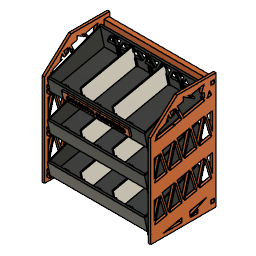
binstack-print-assembly (Autodesk Fusion 360 design; units mm, degrees)
part number: 2026-08-18-20-49-02-766
part number: 2026-08-18-20-49-04-076
part number: 2026-08-18-20-49-04-669
part number: 2026-08-18-20-49-05-390
part number: 2026-08-18-20-49-06-631
part number: 2026-08-18-20-49-07-047
part number: 2026-08-18-20-49-07-130
Autodesk Fusion 360 part; units mm, degrees
sketch "Sketch1" plane through (0, 0, 0) normal (1, 0, 0) x (0, 0, -1) in component "Боковина левая"
  line L0 (0, 15) -> (0, 150)
  line L1 (0, 150) -> (-240, 150)
  line L2 (-240, 150) -> (-240, 70)
  line L3 (-240, 70) -> (-190, 15)
  line L4 (-190, 15) -> (0, 15)
extrude "Extrude1" add sketch "Sketch1" along normal blind 5 from surface at 3 makes body 1 in component "Боковина левая"
sketch "Sketch2" plane through (0, 0, 0) normal (1, 0, 0) x (0, 0, -1) in component "Боковина левая"
  line L0 (-9, 20) -> (-35.5696, 145)
  line L1 (-35.5696, 145) -> (-41.5696, 145)
  line L2 (-41.5696, 145) -> (-15, 20)
  line L3 (-15, 20) -> (-9, 20)
extrude "Extrude2" add sketch "Sketch2" along normal blind 6 from surface at 8 separate body makes body 2 in component "Боковина левая"
sketch "Sketch3" plane through (0, 0, 0) normal (1, 0, 0) x (0, 0, -1) in component "Боковина левая"
  line L0 (-18.2, 20) -> (-44.7696, 145)
  line L1 (-44.7696, 145) -> (-49.7696, 145)
  line L2 (-49.7696, 145) -> (-23.2, 20)
  line L3 (-23.2, 20) -> (-18.2, 20)
extrude "Extrude3" add sketch "Sketch3" along normal blind 6 from surface at 8 separate body makes body 3 in component "Боковина левая"
sketch "Sketch4" plane through (0, 0, 0) normal (1, 0, 0) x (0, 0, -1) in component "Боковина левая"
  line L0 (-16.2753, 26) -> (-17.2753, 28)
  line L1 (-17.2753, 28) -> (-18.3381, 31)
  line L2 (-18.3381, 31) -> (-17.7632, 33)
  line L3 (-17.7632, 33) -> (-16.2753, 26)
extrude "Extrude4" add sketch "Sketch4" along normal blind 6 from surface at 8 separate body makes body 4 in component "Боковина левая"
sketch "Sketch5" plane through (0, 0, 0) normal (1, 0, 0) x (0, 0, -1) in component "Боковина левая"
  line L0 (-84, 20) -> (-110.5696, 145)
  line L1 (-110.5696, 145) -> (-116.5696, 145)
  line L2 (-116.5696, 145) -> (-90, 20)
  line L3 (-90, 20) -> (-84, 20)
extrude "Extrude5" add sketch "Sketch5" along normal blind 6 from surface at 8 separate body makes body 5 in component "Боковина левая"
sketch "Sketch6" plane through (0, 0, 0) normal (1, 0, 0) x (0, 0, -1) in component "Боковина левая"
  line L0 (-93.2, 20) -> (-119.7696, 145)
  line L1 (-119.7696, 145) -> (-124.7696, 145)
  line L2 (-124.7696, 145) -> (-98.2, 20)
  line L3 (-98.2, 20) -> (-93.2, 20)
extrude "Extrude6" add sketch "Sketch6" along normal blind 6 from surface at 8 separate body makes body 6 in component "Боковина левая"
sketch "Sketch7" plane through (0, 0, 0) normal (1, 0, 0) x (0, 0, -1) in component "Боковина левая"
  line L0 (-91.2753, 26) -> (-92.2753, 28)
  line L1 (-92.2753, 28) -> (-93.3381, 31)
  line L2 (-93.3381, 31) -> (-92.7632, 33)
  line L3 (-92.7632, 33) -> (-91.2753, 26)
extrude "Extrude7" add sketch "Sketch7" along normal blind 6 from surface at 8 separate body makes body 7 in component "Боковина левая"
sketch "Sketch8" plane through (0, 0, 0) normal (1, 0, 0) x (0, 0, -1) in component "Боковина левая"
  line L0 (-159, 20) -> (-185.5696, 145)
  line L1 (-185.5696, 145) -> (-191.5696, 145)
  line L2 (-191.5696, 145) -> (-165, 20)
  line L3 (-165, 20) -> (-159, 20)
extrude "Extrude8" add sketch "Sketch8" along normal blind 6 from surface at 8 separate body makes body 8 in component "Боковина левая"
sketch "Sketch9" plane through (0, 0, 0) normal (1, 0, 0) x (0, 0, -1) in component "Боковина левая"
  line L0 (-168.2, 20) -> (-194.7696, 145)
  line L1 (-194.7696, 145) -> (-199.7696, 145)
  line L2 (-199.7696, 145) -> (-173.2, 20)
  line L3 (-173.2, 20) -> (-168.2, 20)
extrude "Extrude9" add sketch "Sketch9" along normal blind 6 from surface at 8 separate body makes body 9 in component "Боковина левая"
sketch "Sketch10" plane through (0, 0, 0) normal (1, 0, 0) x (0, 0, -1) in component "Боковина левая"
  line L0 (-166.2753, 26) -> (-167.2753, 28)
  line L1 (-167.2753, 28) -> (-168.3381, 31)
  line L2 (-168.3381, 31) -> (-167.7632, 33)
  line L3 (-167.7632, 33) -> (-166.2753, 26)
extrude "Extrude10" add sketch "Sketch10" along normal blind 6 from surface at 8 separate body makes body 10 in component "Боковина левая"
combine "Combine1" operation add target body 1 tool bodies 2 3 4 5 6 7 8 9 10 in component "Боковина левая"
sketch "Sketch11" plane through (0, 0, 0) normal (1, 0, 0) x (0, 0, -1) in component "Боковина левая"
  line L0 (-10.5, 139.5) -> (-10.5, 146.5)
  line L1 (-10.5, 146.5) -> (-17.5, 146.5)
  line L2 (-17.5, 146.5) -> (-17.5, 139.5)
  line L3 (-17.5, 139.5) -> (-10.5, 139.5)
extrude "Extrude11" cut sketch "Sketch11" along normal blind 30 from surface at -2 bodies 1 in component "Боковина левая"
sketch "Sketch12" plane through (0, 0, 0) normal (1, 0, 0) x (0, 0, -1) in component "Боковина левая"
  line L0 (-222.5, 139.5) -> (-222.5, 146.5)
  line L1 (-222.5, 146.5) -> (-229.5, 146.5)
  line L2 (-229.5, 146.5) -> (-229.5, 139.5)
  line L3 (-229.5, 139.5) -> (-222.5, 139.5)
extrude "Extrude12" cut sketch "Sketch12" along normal blind 30 from surface at -2 bodies 1 in component "Боковина левая"
sketch "Sketch13" plane through (0, 0, 0) normal (1, 0, 0) x (0, 0, -1) in component "Боковина левая"
  line L0 (-31.0484, 23.6788) -> (-36.4457, 49.0712)
  line L1 (-36.4457, 49.0712) -> (-77.3478, 36.375)
  line L2 (-77.3478, 36.375) -> (-31.0484, 23.6788)
  line L3 (-37.5845, 54.4288) -> (-42.9818, 79.8212)
  line L4 (-42.9818, 79.8212) -> (-83.8839, 67.125)
  line L5 (-83.8839, 67.125) -> (-37.5845, 54.4288)
  line L6 (-44.1206, 85.1788) -> (-49.5179, 110.5712)
  line L7 (-49.5179, 110.5712) -> (-90.42, 97.875)
  line L8 (-90.42, 97.875) -> (-44.1206, 85.1788)
  line L9 (-50.6567, 115.9288) -> (-56.054, 141.3212)
  line L10 (-56.054, 141.3212) -> (-96.9561, 128.625)
  line L11 (-96.9561, 128.625) -> (-50.6567, 115.9288)
  line L12 (-80.9836, 39.0538) -> (-86.3809, 64.4462)
  line L13 (-86.3809, 64.4462) -> (-40.0815, 51.75)
  line L14 (-40.0815, 51.75) -> (-80.9836, 39.0538)
  line L15 (-87.5197, 69.8038) -> (-92.917, 95.1962)
  line L16 (-92.917, 95.1962) -> (-46.6176, 82.5)
  line L17 (-46.6176, 82.5) -> (-87.5197, 69.8038)
  line L18 (-94.0558, 100.5538) -> (-99.4532, 125.9462)
  line L19 (-99.4532, 125.9462) -> (-53.1537, 113.25)
  line L20 (-53.1537, 113.25) -> (-94.0558, 100.5538)
  line L21 (-38.7362, 22.5992) -> (-75.0606, 22.5992)
  line L22 (-75.0606, 22.5992) -> (-77.3089, 33.1766)
  line L23 (-77.3089, 33.1766) -> (-38.7362, 22.5992)
  line L24 (-63.6735, 142.48) -> (-100.8141, 142.48)
  line L25 (-100.8141, 142.48) -> (-98.5153, 131.6649)
  line L26 (-98.5153, 131.6649) -> (-63.6735, 142.48)
  line L27 (-106.0484, 23.6788) -> (-111.4457, 49.0712)
  line L28 (-111.4457, 49.0712) -> (-152.3478, 36.375)
  line L29 (-152.3478, 36.375) -> (-106.0484, 23.6788)
  line L30 (-112.5845, 54.4288) -> (-117.9818, 79.8212)
  line L31 (-117.9818, 79.8212) -> (-158.8839, 67.125)
  line L32 (-158.8839, 67.125) -> (-112.5845, 54.4288)
  line L33 (-119.1206, 85.1788) -> (-124.5179, 110.5712)
  line L34 (-124.5179, 110.5712) -> (-165.42, 97.875)
  line L35 (-165.42, 97.875) -> (-119.1206, 85.1788)
  line L36 (-125.6567, 115.9288) -> (-131.054, 141.3212)
  line L37 (-131.054, 141.3212) -> (-171.9561, 128.625)
  line L38 (-171.9561, 128.625) -> (-125.6567, 115.9288)
  line L39 (-155.9836, 39.0538) -> (-161.3809, 64.4462)
  line L40 (-161.3809, 64.4462) -> (-115.0815, 51.75)
  line L41 (-115.0815, 51.75) -> (-155.9836, 39.0538)
  line L42 (-162.5197, 69.8038) -> (-167.917, 95.1962)
  line L43 (-167.917, 95.1962) -> (-121.6176, 82.5)
  line L44 (-121.6176, 82.5) -> (-162.5197, 69.8038)
  line L45 (-169.0558, 100.5538) -> (-174.4532, 125.9462)
  line L46 (-174.4532, 125.9462) -> (-128.1537, 113.25)
  line L47 (-128.1537, 113.25) -> (-169.0558, 100.5538)
  line L48 (-113.7362, 22.5992) -> (-150.0606, 22.5992)
  line L49 (-150.0606, 22.5992) -> (-152.3089, 33.1766)
  line L50 (-152.3089, 33.1766) -> (-113.7362, 22.5992)
  line L51 (-138.6735, 142.48) -> (-175.8141, 142.48)
  line L52 (-175.8141, 142.48) -> (-173.5153, 131.6649)
  line L53 (-173.5153, 131.6649) -> (-138.6735, 142.48)
  line L54 (-180.386, 24.1097) -> (-182.3321, 33.2653)
  line L55 (-182.3321, 33.2653) -> (-191.5717, 28.6875)
  line L56 (-191.5717, 28.6875) -> (-180.386, 24.1097)
  line L57 (-183.654, 39.4847) -> (-185.6001, 48.6403)
  line L58 (-185.6001, 48.6403) -> (-194.8398, 44.0625)
  line L59 (-194.8398, 44.0625) -> (-183.654, 39.4847)
  line L60 (-185.3055, 36.375) -> (-196.4912, 40.9528)
  line L61 (-196.4912, 40.9528) -> (-194.5451, 31.7972)
  line L62 (-194.5451, 31.7972) -> (-185.3055, 36.375)
  line L63 (-186.9221, 54.8597) -> (-192.1362, 79.3903)
  line L64 (-192.1362, 79.3903) -> (-216.8918, 67.125)
  line L65 (-216.8918, 67.125) -> (-186.9221, 54.8597)
  line L66 (-193.4582, 85.6097) -> (-198.6724, 110.1403)
  line L67 (-198.6724, 110.1403) -> (-223.428, 97.875)
  line L68 (-223.428, 97.875) -> (-193.4582, 85.6097)
  line L69 (-199.9943, 116.3597) -> (-201.9404, 125.5153)
  line L70 (-201.9404, 125.5153) -> (-211.18, 120.9375)
  line L71 (-211.18, 120.9375) -> (-199.9943, 116.3597)
  line L72 (-203.2624, 131.7347) -> (-205.2085, 140.8903)
  line L73 (-205.2085, 140.8903) -> (-214.4481, 136.3125)
  line L74 (-214.4481, 136.3125) -> (-203.2624, 131.7347)
  line L75 (-216.5972, 54.8597) -> (-218.5433, 64.0153)
  line L76 (-218.5433, 64.0153) -> (-207.3576, 59.4375)
  line L77 (-207.3576, 59.4375) -> (-216.5972, 54.8597)
  line L78 (-197.8132, 47.1722) -> (-199.7593, 56.3278)
  line L79 (-199.7593, 56.3278) -> (-188.5736, 51.75)
  line L80 (-188.5736, 51.75) -> (-197.8132, 47.1722)
  line L81 (-213.6238, 51.75) -> (-204.3842, 56.3278)
  line L82 (-204.3842, 56.3278) -> (-202.4381, 47.1722)
  line L83 (-202.4381, 47.1722) -> (-213.6238, 51.75)
  line L84 (-219.8653, 70.2347) -> (-225.0794, 94.7653)
  line L85 (-225.0794, 94.7653) -> (-195.1097, 82.5)
  line L86 (-195.1097, 82.5) -> (-219.8653, 70.2347)
  line L87 (-226.4014, 100.9847) -> (-231.6155, 125.5153)
  line L88 (-231.6155, 125.5153) -> (-201.6458, 113.25)
  line L89 (-201.6458, 113.25) -> (-226.4014, 100.9847)
  line L90 (-7.4997, 41.3524) -> (-7.4997, 79.3238)
  line L91 (-7.4997, 79.3238) -> (-16.0293, 79.3238)
  line L92 (-16.0293, 79.3238) -> (-7.4997, 41.3524)
  line L93 (-7.7256, 97.1983) -> (-7.7256, 112.4009)
  line L94 (-7.7256, 112.4009) -> (-15.0147, 112.4009)
  line L95 (-15.0147, 112.4009) -> (-7.7256, 97.1983)
  line L96 (-10.4709, 95.9903) -> (-19.5534, 95.9903)
  line L97 (-19.5534, 95.9903) -> (-26.7865, 130.0194)
  line L98 (-26.7865, 130.0194) -> (-10.4709, 95.9903)
  line L99 (-181.1006, 31.0194) -> (-188.5277, 65.9611)
  line L100 (-188.5277, 65.9611) -> (-191.9491, 31.0194)
  line L101 (-191.9491, 31.0194) -> (-181.1006, 31.0194)
  line L102 (-191.1748, 72.6899) -> (-212.3291, 72.6899)
  line L103 (-212.3291, 72.6899) -> (-195.0983, 32.6201)
  line L104 (-195.0983, 32.6201) -> (-191.1748, 72.6899)
  line L105 (-192.5, 82.4034) -> (-202.0204, 127.1932)
  line L106 (-202.0204, 127.1932) -> (-230.4393, 82.4034)
  line L107 (-230.4393, 82.4034) -> (-192.5, 82.4034)
  line L108 (-206.5204, 125.9619) -> (-215.9652, 125.9619)
  line L109 (-215.9652, 125.9619) -> (-228.0207, 92.0761)
  line L110 (-228.0207, 92.0761) -> (-206.5204, 125.9619)
extrude "Extrude13" cut sketch "Sketch13" along normal blind 9 from surface at 1 bodies 1 in component "Боковина левая"
sketch "Sketch1 (2)" plane through (0, 0, 0) normal (1, 0, 0) x (0, 0, -1) in component "Боковина правая"
  line L0 (0, 15) -> (0, 150)
  line L1 (0, 150) -> (-240, 150)
  line L2 (-240, 150) -> (-240, 70)
  line L3 (-240, 70) -> (-190, 15)
  line L4 (-190, 15) -> (0, 15)
extrude "Extrude1'" add sketch "Sketch1 (2)" along normal blind 5 from surface at 6 separate body makes body 11 in component "Боковина правая"
sketch "Sketch2 (2)" plane through (0, 0, 0) normal (1, 0, 0) x (0, 0, -1) in component "Боковина правая"
  line L0 (-9, 20) -> (-35.5696, 145)
  line L1 (-35.5696, 145) -> (-41.5696, 145)
  line L2 (-41.5696, 145) -> (-15, 20)
  line L3 (-15, 20) -> (-9, 20)
extrude "Extrude2'" add sketch "Sketch2 (2)" along normal blind 6 separate body makes body 12 in component "Боковина правая"
sketch "Sketch3 (2)" plane through (0, 0, 0) normal (1, 0, 0) x (0, 0, -1) in component "Боковина правая"
  line L0 (-18.2, 20) -> (-44.7696, 145)
  line L1 (-44.7696, 145) -> (-49.7696, 145)
  line L2 (-49.7696, 145) -> (-23.2, 20)
  line L3 (-23.2, 20) -> (-18.2, 20)
extrude "Extrude3'" add sketch "Sketch3 (2)" along normal blind 6 separate body makes body 13 in component "Боковина правая"
sketch "Sketch4 (2)" plane through (0, 0, 0) normal (1, 0, 0) x (0, 0, -1) in component "Боковина правая"
  line L0 (-16.2753, 26) -> (-17.2753, 28)
  line L1 (-17.2753, 28) -> (-18.3381, 31)
  line L2 (-18.3381, 31) -> (-17.7632, 33)
  line L3 (-17.7632, 33) -> (-16.2753, 26)
extrude "Extrude4'" add sketch "Sketch4 (2)" along normal blind 6 separate body makes body 14 in component "Боковина правая"
sketch "Sketch5 (2)" plane through (0, 0, 0) normal (1, 0, 0) x (0, 0, -1) in component "Боковина правая"
  line L0 (-84, 20) -> (-110.5696, 145)
  line L1 (-110.5696, 145) -> (-116.5696, 145)
  line L2 (-116.5696, 145) -> (-90, 20)
  line L3 (-90, 20) -> (-84, 20)
extrude "Extrude5'" add sketch "Sketch5 (2)" along normal blind 6 separate body makes body 15 in component "Боковина правая"
sketch "Sketch6 (2)" plane through (0, 0, 0) normal (1, 0, 0) x (0, 0, -1) in component "Боковина правая"
  line L0 (-93.2, 20) -> (-119.7696, 145)
  line L1 (-119.7696, 145) -> (-124.7696, 145)
  line L2 (-124.7696, 145) -> (-98.2, 20)
  line L3 (-98.2, 20) -> (-93.2, 20)
extrude "Extrude6'" add sketch "Sketch6 (2)" along normal blind 6 separate body makes body 16 in component "Боковина правая"
sketch "Sketch7 (2)" plane through (0, 0, 0) normal (1, 0, 0) x (0, 0, -1) in component "Боковина правая"
  line L0 (-91.2753, 26) -> (-92.2753, 28)
  line L1 (-92.2753, 28) -> (-93.3381, 31)
  line L2 (-93.3381, 31) -> (-92.7632, 33)
  line L3 (-92.7632, 33) -> (-91.2753, 26)
extrude "Extrude7'" add sketch "Sketch7 (2)" along normal blind 6 separate body makes body 17 in component "Боковина правая"
sketch "Sketch8 (2)" plane through (0, 0, 0) normal (1, 0, 0) x (0, 0, -1) in component "Боковина правая"
  line L0 (-159, 20) -> (-185.5696, 145)
  line L1 (-185.5696, 145) -> (-191.5696, 145)
  line L2 (-191.5696, 145) -> (-165, 20)
  line L3 (-165, 20) -> (-159, 20)
extrude "Extrude8'" add sketch "Sketch8 (2)" along normal blind 6 separate body makes body 18 in component "Боковина правая"
sketch "Sketch9 (2)" plane through (0, 0, 0) normal (1, 0, 0) x (0, 0, -1) in component "Боковина правая"
  line L0 (-168.2, 20) -> (-194.7696, 145)
  line L1 (-194.7696, 145) -> (-199.7696, 145)
  line L2 (-199.7696, 145) -> (-173.2, 20)
  line L3 (-173.2, 20) -> (-168.2, 20)
extrude "Extrude9'" add sketch "Sketch9 (2)" along normal blind 6 separate body makes body 19 in component "Боковина правая"
sketch "Sketch10 (2)" plane through (0, 0, 0) normal (1, 0, 0) x (0, 0, -1) in component "Боковина правая"
  line L0 (-166.2753, 26) -> (-167.2753, 28)
  line L1 (-167.2753, 28) -> (-168.3381, 31)
  line L2 (-168.3381, 31) -> (-167.7632, 33)
  line L3 (-167.7632, 33) -> (-166.2753, 26)
extrude "Extrude10'" add sketch "Sketch10 (2)" along normal blind 6 separate body makes body 20 in component "Боковина правая"
combine "Combine1'" operation add target body 11 tool bodies 12 13 14 15 16 17 18 19 20 in component "Боковина правая"
sketch "Sketch11 (2)" plane through (0, 0, 0) normal (1, 0, 0) x (0, 0, -1) in component "Боковина правая"
  line L0 (-10.5, 139.5) -> (-10.5, 146.5)
  line L1 (-10.5, 146.5) -> (-17.5, 146.5)
  line L2 (-17.5, 146.5) -> (-17.5, 139.5)
  line L3 (-17.5, 139.5) -> (-10.5, 139.5)
extrude "Extrude11'" cut sketch "Sketch11 (2)" along normal blind 30 from surface at -2 bodies 11 in component "Боковина правая"
sketch "Sketch12 (2)" plane through (0, 0, 0) normal (1, 0, 0) x (0, 0, -1) in component "Боковина правая"
  line L0 (-222.5, 139.5) -> (-222.5, 146.5)
  line L1 (-222.5, 146.5) -> (-229.5, 146.5)
  line L2 (-229.5, 146.5) -> (-229.5, 139.5)
  line L3 (-229.5, 139.5) -> (-222.5, 139.5)
extrude "Extrude12'" cut sketch "Sketch12 (2)" along normal blind 30 from surface at -2 bodies 11 in component "Боковина правая"
sketch "Sketch13 (2)" plane through (0, 0, 0) normal (1, 0, 0) x (0, 0, -1) in component "Боковина правая"
  line L0 (-31.0484, 23.6788) -> (-36.4457, 49.0712)
  line L1 (-36.4457, 49.0712) -> (-77.3478, 36.375)
  line L2 (-77.3478, 36.375) -> (-31.0484, 23.6788)
  line L3 (-37.5845, 54.4288) -> (-42.9818, 79.8212)
  line L4 (-42.9818, 79.8212) -> (-83.8839, 67.125)
  line L5 (-83.8839, 67.125) -> (-37.5845, 54.4288)
  line L6 (-44.1206, 85.1788) -> (-49.5179, 110.5712)
  line L7 (-49.5179, 110.5712) -> (-90.42, 97.875)
  line L8 (-90.42, 97.875) -> (-44.1206, 85.1788)
  line L9 (-50.6567, 115.9288) -> (-56.054, 141.3212)
  line L10 (-56.054, 141.3212) -> (-96.9561, 128.625)
  line L11 (-96.9561, 128.625) -> (-50.6567, 115.9288)
  line L12 (-80.9836, 39.0538) -> (-86.3809, 64.4462)
  line L13 (-86.3809, 64.4462) -> (-40.0815, 51.75)
  line L14 (-40.0815, 51.75) -> (-80.9836, 39.0538)
  line L15 (-87.5197, 69.8038) -> (-92.917, 95.1962)
  line L16 (-92.917, 95.1962) -> (-46.6176, 82.5)
  line L17 (-46.6176, 82.5) -> (-87.5197, 69.8038)
  line L18 (-94.0558, 100.5538) -> (-99.4532, 125.9462)
  line L19 (-99.4532, 125.9462) -> (-53.1537, 113.25)
  line L20 (-53.1537, 113.25) -> (-94.0558, 100.5538)
  line L21 (-38.7362, 22.5992) -> (-75.0606, 22.5992)
  line L22 (-75.0606, 22.5992) -> (-77.3089, 33.1766)
  line L23 (-77.3089, 33.1766) -> (-38.7362, 22.5992)
  line L24 (-63.6735, 142.48) -> (-100.8141, 142.48)
  line L25 (-100.8141, 142.48) -> (-98.5153, 131.6649)
  line L26 (-98.5153, 131.6649) -> (-63.6735, 142.48)
  line L27 (-106.0484, 23.6788) -> (-111.4457, 49.0712)
  line L28 (-111.4457, 49.0712) -> (-152.3478, 36.375)
  line L29 (-152.3478, 36.375) -> (-106.0484, 23.6788)
  line L30 (-112.5845, 54.4288) -> (-117.9818, 79.8212)
  line L31 (-117.9818, 79.8212) -> (-158.8839, 67.125)
  line L32 (-158.8839, 67.125) -> (-112.5845, 54.4288)
  line L33 (-119.1206, 85.1788) -> (-124.5179, 110.5712)
  line L34 (-124.5179, 110.5712) -> (-165.42, 97.875)
  line L35 (-165.42, 97.875) -> (-119.1206, 85.1788)
  line L36 (-125.6567, 115.9288) -> (-131.054, 141.3212)
  line L37 (-131.054, 141.3212) -> (-171.9561, 128.625)
  line L38 (-171.9561, 128.625) -> (-125.6567, 115.9288)
  line L39 (-155.9836, 39.0538) -> (-161.3809, 64.4462)
  line L40 (-161.3809, 64.4462) -> (-115.0815, 51.75)
  line L41 (-115.0815, 51.75) -> (-155.9836, 39.0538)
  line L42 (-162.5197, 69.8038) -> (-167.917, 95.1962)
  line L43 (-167.917, 95.1962) -> (-121.6176, 82.5)
  line L44 (-121.6176, 82.5) -> (-162.5197, 69.8038)
  line L45 (-169.0558, 100.5538) -> (-174.4532, 125.9462)
  line L46 (-174.4532, 125.9462) -> (-128.1537, 113.25)
  line L47 (-128.1537, 113.25) -> (-169.0558, 100.5538)
  line L48 (-113.7362, 22.5992) -> (-150.0606, 22.5992)
  line L49 (-150.0606, 22.5992) -> (-152.3089, 33.1766)
  line L50 (-152.3089, 33.1766) -> (-113.7362, 22.5992)
  line L51 (-138.6735, 142.48) -> (-175.8141, 142.48)
  line L52 (-175.8141, 142.48) -> (-173.5153, 131.6649)
  line L53 (-173.5153, 131.6649) -> (-138.6735, 142.48)
  line L54 (-180.386, 24.1097) -> (-182.3321, 33.2653)
  line L55 (-182.3321, 33.2653) -> (-191.5717, 28.6875)
  line L56 (-191.5717, 28.6875) -> (-180.386, 24.1097)
  line L57 (-183.654, 39.4847) -> (-185.6001, 48.6403)
  line L58 (-185.6001, 48.6403) -> (-194.8398, 44.0625)
  line L59 (-194.8398, 44.0625) -> (-183.654, 39.4847)
  line L60 (-185.3055, 36.375) -> (-196.4912, 40.9528)
  line L61 (-196.4912, 40.9528) -> (-194.5451, 31.7972)
  line L62 (-194.5451, 31.7972) -> (-185.3055, 36.375)
  line L63 (-186.9221, 54.8597) -> (-192.1362, 79.3903)
  line L64 (-192.1362, 79.3903) -> (-216.8918, 67.125)
  line L65 (-216.8918, 67.125) -> (-186.9221, 54.8597)
  line L66 (-193.4582, 85.6097) -> (-198.6724, 110.1403)
  line L67 (-198.6724, 110.1403) -> (-223.428, 97.875)
  line L68 (-223.428, 97.875) -> (-193.4582, 85.6097)
  line L69 (-199.9943, 116.3597) -> (-201.9404, 125.5153)
  line L70 (-201.9404, 125.5153) -> (-211.18, 120.9375)
  line L71 (-211.18, 120.9375) -> (-199.9943, 116.3597)
  line L72 (-203.2624, 131.7347) -> (-205.2085, 140.8903)
  line L73 (-205.2085, 140.8903) -> (-214.4481, 136.3125)
  line L74 (-214.4481, 136.3125) -> (-203.2624, 131.7347)
  line L75 (-216.5972, 54.8597) -> (-218.5433, 64.0153)
  line L76 (-218.5433, 64.0153) -> (-207.3576, 59.4375)
  line L77 (-207.3576, 59.4375) -> (-216.5972, 54.8597)
  line L78 (-197.8132, 47.1722) -> (-199.7593, 56.3278)
  line L79 (-199.7593, 56.3278) -> (-188.5736, 51.75)
  line L80 (-188.5736, 51.75) -> (-197.8132, 47.1722)
  line L81 (-213.6238, 51.75) -> (-204.3842, 56.3278)
  line L82 (-204.3842, 56.3278) -> (-202.4381, 47.1722)
  line L83 (-202.4381, 47.1722) -> (-213.6238, 51.75)
  line L84 (-219.8653, 70.2347) -> (-225.0794, 94.7653)
  line L85 (-225.0794, 94.7653) -> (-195.1097, 82.5)
  line L86 (-195.1097, 82.5) -> (-219.8653, 70.2347)
  line L87 (-226.4014, 100.9847) -> (-231.6155, 125.5153)
  line L88 (-231.6155, 125.5153) -> (-201.6458, 113.25)
  line L89 (-201.6458, 113.25) -> (-226.4014, 100.9847)
  line L90 (-7.4997, 41.3524) -> (-7.4997, 79.3238)
  line L91 (-7.4997, 79.3238) -> (-16.0293, 79.3238)
  line L92 (-16.0293, 79.3238) -> (-7.4997, 41.3524)
  line L93 (-7.7256, 97.1983) -> (-7.7256, 112.4009)
  line L94 (-7.7256, 112.4009) -> (-15.0147, 112.4009)
  line L95 (-15.0147, 112.4009) -> (-7.7256, 97.1983)
  line L96 (-10.4709, 95.9903) -> (-19.5534, 95.9903)
  line L97 (-19.5534, 95.9903) -> (-26.7865, 130.0194)
  line L98 (-26.7865, 130.0194) -> (-10.4709, 95.9903)
  line L99 (-181.1006, 31.0194) -> (-188.5277, 65.9611)
  line L100 (-188.5277, 65.9611) -> (-191.9491, 31.0194)
  line L101 (-191.9491, 31.0194) -> (-181.1006, 31.0194)
  line L102 (-191.1748, 72.6899) -> (-212.3291, 72.6899)
  line L103 (-212.3291, 72.6899) -> (-195.0983, 32.6201)
  line L104 (-195.0983, 32.6201) -> (-191.1748, 72.6899)
  line L105 (-192.5, 82.4034) -> (-202.0204, 127.1932)
  line L106 (-202.0204, 127.1932) -> (-230.4393, 82.4034)
  line L107 (-230.4393, 82.4034) -> (-192.5, 82.4034)
  line L108 (-206.5204, 125.9619) -> (-215.9652, 125.9619)
  line L109 (-215.9652, 125.9619) -> (-228.0207, 92.0761)
  line L110 (-228.0207, 92.0761) -> (-206.5204, 125.9619)
extrude "Extrude13'" cut sketch "Sketch13 (2)" along normal blind 9 from surface at 4 bodies 11 in component "Боковина правая"
sketch "Sketch1 (3)" plane through (0, 0, 0) normal (0, 0, 1) x (1, 0, 0) in component "Лоток"
  line L0 (-6, 0) -> (207, 0)
  line L1 (207, 0) -> (207, 117)
  line L2 (207, 117) -> (-6, 117)
  line L3 (-6, 117) -> (-6, 0)
extrude "Extrude1''" add sketch "Sketch1 (3)" along normal blind 2.4 separate body makes body 21 in component "Лоток"
sketch "Sketch2 (3)" plane through (0, 0, 0) normal (0, 0, 1) x (1, 0, 0) in component "Лоток"
  line L0 (0, 0) -> (201, 0)
  line L1 (201, 0) -> (201, 4)
  line L2 (201, 4) -> (0, 4)
  line L3 (0, 4) -> (0, 0)
extrude "Extrude2''" add sketch "Sketch2 (3)" along normal blind 28 separate body makes body 22 in component "Лоток"
sketch "Sketch3 (3)" plane through (0, 0, 0) normal (0, 0, 1) x (1, 0, 0) in component "Лоток"
  line L0 (0, 113) -> (201, 113)
  line L1 (201, 113) -> (201, 117)
  line L2 (201, 117) -> (0, 117)
  line L3 (0, 117) -> (0, 113)
extrude "Extrude3''" add sketch "Sketch3 (3)" along normal blind 45 separate body makes body 23 in component "Лоток"
sketch "Sketch4 (3)" plane through (0, 0, 0) normal (1, 0, 0) x (0, 0, -1) in component "Лоток"
  line L0 (0, 0) -> (0, 117)
  line L1 (0, 117) -> (-45, 117)
  line L2 (-45, 117) -> (-28, 0)
  line L3 (-28, 0) -> (0, 0)
extrude "Extrude4''" add sketch "Sketch4 (3)" along normal blind 2 separate body makes body 24 in component "Лоток"
sketch "Sketch5 (3)" plane through (0, 0, 0) normal (1, 0, 0) x (0, 0, -1) in component "Лоток"
  line L0 (0, 0) -> (0, 117)
  line L1 (0, 117) -> (-45, 117)
  line L2 (-45, 117) -> (-28, 0)
  line L3 (-28, 0) -> (0, 0)
extrude "Extrude5''" add sketch "Sketch5 (3)" along normal blind 2 from surface at 199 separate body makes body 25 in component "Лоток"
sketch "Sketch6 (3)" plane through (0, 0, 0) normal (0, 0, 1) x (1, 0, 0) in component "Лоток"
  line L0 (31.4, 4) -> (33.4, 4)
  line L1 (33.4, 4) -> (33.4, 6)
  line L2 (33.4, 6) -> (31.4, 6)
  line L3 (31.4, 6) -> (31.4, 4)
extrude "Extrude6''" add sketch "Sketch6 (3)" along normal blind 25.6 from surface at 2.4 separate body makes body 26 in component "Лоток"
sketch "Sketch7 (3)" plane through (0, 0, 0) normal (0, 0, 1) x (1, 0, 0) in component "Лоток"
  line L0 (31.4, 111) -> (33.4, 111)
  line L1 (33.4, 111) -> (33.4, 113)
  line L2 (33.4, 113) -> (31.4, 113)
  line L3 (31.4, 113) -> (31.4, 111)
extrude "Extrude7''" add sketch "Sketch7 (3)" along normal blind 42.6 from surface at 2.4 separate body makes body 27 in component "Лоток"
sketch "Sketch8 (3)" plane through (0, 0, 0) normal (0, 0, 1) x (1, 0, 0) in component "Лоток"
  line L0 (36.6, 4) -> (38.6, 4)
  line L1 (38.6, 4) -> (38.6, 6)
  line L2 (38.6, 6) -> (36.6, 6)
  line L3 (36.6, 6) -> (36.6, 4)
extrude "Extrude8''" add sketch "Sketch8 (3)" along normal blind 25.6 from surface at 2.4 separate body makes body 28 in component "Лоток"
sketch "Sketch9 (3)" plane through (0, 0, 0) normal (0, 0, 1) x (1, 0, 0) in component "Лоток"
  line L0 (36.6, 111) -> (38.6, 111)
  line L1 (38.6, 111) -> (38.6, 113)
  line L2 (38.6, 113) -> (36.6, 113)
  line L3 (36.6, 113) -> (36.6, 111)
extrude "Extrude9''" add sketch "Sketch9 (3)" along normal blind 42.6 from surface at 2.4 separate body makes body 29 in component "Лоток"
sketch "Sketch10 (3)" plane through (0, 0, 0) normal (0, 0, 1) x (1, 0, 0) in component "Лоток"
  line L0 (64.4, 4) -> (66.4, 4)
  line L1 (66.4, 4) -> (66.4, 6)
  line L2 (66.4, 6) -> (64.4, 6)
  line L3 (64.4, 6) -> (64.4, 4)
extrude "Extrude10''" add sketch "Sketch10 (3)" along normal blind 25.6 from surface at 2.4 separate body makes body 30 in component "Лоток"
sketch "Sketch11 (3)" plane through (0, 0, 0) normal (0, 0, 1) x (1, 0, 0) in component "Лоток"
  line L0 (64.4, 111) -> (66.4, 111)
  line L1 (66.4, 111) -> (66.4, 113)
  line L2 (66.4, 113) -> (64.4, 113)
  line L3 (64.4, 113) -> (64.4, 111)
extrude "Extrude11''" add sketch "Sketch11 (3)" along normal blind 42.6 from surface at 2.4 separate body makes body 31 in component "Лоток"
sketch "Sketch12 (3)" plane through (0, 0, 0) normal (0, 0, 1) x (1, 0, 0) in component "Лоток"
  line L0 (69.6, 4) -> (71.6, 4)
  line L1 (71.6, 4) -> (71.6, 6)
  line L2 (71.6, 6) -> (69.6, 6)
  line L3 (69.6, 6) -> (69.6, 4)
extrude "Extrude12''" add sketch "Sketch12 (3)" along normal blind 25.6 from surface at 2.4 separate body makes body 32 in component "Лоток"
sketch "Sketch13 (3)" plane through (0, 0, 0) normal (0, 0, 1) x (1, 0, 0) in component "Лоток"
  line L0 (69.6, 111) -> (71.6, 111)
  line L1 (71.6, 111) -> (71.6, 113)
  line L2 (71.6, 113) -> (69.6, 113)
  line L3 (69.6, 113) -> (69.6, 111)
extrude "Extrude13''" add sketch "Sketch13 (3)" along normal blind 42.6 from surface at 2.4 separate body makes body 33 in component "Лоток"
sketch "Sketch14" plane through (0, 0, 0) normal (0, 0, 1) x (1, 0, 0) in component "Лоток"
  line L0 (97.4, 4) -> (99.4, 4)
  line L1 (99.4, 4) -> (99.4, 6)
  line L2 (99.4, 6) -> (97.4, 6)
  line L3 (97.4, 6) -> (97.4, 4)
extrude "Extrude14" add sketch "Sketch14" along normal blind 25.6 from surface at 2.4 separate body makes body 34 in component "Лоток"
sketch "Sketch15" plane through (0, 0, 0) normal (0, 0, 1) x (1, 0, 0) in component "Лоток"
  line L0 (97.4, 111) -> (99.4, 111)
  line L1 (99.4, 111) -> (99.4, 113)
  line L2 (99.4, 113) -> (97.4, 113)
  line L3 (97.4, 113) -> (97.4, 111)
extrude "Extrude15" add sketch "Sketch15" along normal blind 42.6 from surface at 2.4 separate body makes body 35 in component "Лоток"
sketch "Sketch16" plane through (0, 0, 0) normal (0, 0, 1) x (1, 0, 0) in component "Лоток"
  line L0 (102.6, 4) -> (104.6, 4)
  line L1 (104.6, 4) -> (104.6, 6)
  line L2 (104.6, 6) -> (102.6, 6)
  line L3 (102.6, 6) -> (102.6, 4)
extrude "Extrude16" add sketch "Sketch16" along normal blind 25.6 from surface at 2.4 separate body makes body 36 in component "Лоток"
sketch "Sketch17" plane through (0, 0, 0) normal (0, 0, 1) x (1, 0, 0) in component "Лоток"
  line L0 (102.6, 111) -> (104.6, 111)
  line L1 (104.6, 111) -> (104.6, 113)
  line L2 (104.6, 113) -> (102.6, 113)
  line L3 (102.6, 113) -> (102.6, 111)
extrude "Extrude17" add sketch "Sketch17" along normal blind 42.6 from surface at 2.4 separate body makes body 37 in component "Лоток"
sketch "Sketch18" plane through (0, 0, 0) normal (0, 0, 1) x (1, 0, 0) in component "Лоток"
  line L0 (130.4, 4) -> (132.4, 4)
  line L1 (132.4, 4) -> (132.4, 6)
  line L2 (132.4, 6) -> (130.4, 6)
  line L3 (130.4, 6) -> (130.4, 4)
extrude "Extrude18" add sketch "Sketch18" along normal blind 25.6 from surface at 2.4 separate body makes body 38 in component "Лоток"
sketch "Sketch19" plane through (0, 0, 0) normal (0, 0, 1) x (1, 0, 0) in component "Лоток"
  line L0 (130.4, 111) -> (132.4, 111)
  line L1 (132.4, 111) -> (132.4, 113)
  line L2 (132.4, 113) -> (130.4, 113)
  line L3 (130.4, 113) -> (130.4, 111)
extrude "Extrude19" add sketch "Sketch19" along normal blind 42.6 from surface at 2.4 separate body makes body 39 in component "Лоток"
sketch "Sketch20" plane through (0, 0, 0) normal (0, 0, 1) x (1, 0, 0) in component "Лоток"
  line L0 (135.6, 4) -> (137.6, 4)
  line L1 (137.6, 4) -> (137.6, 6)
  line L2 (137.6, 6) -> (135.6, 6)
  line L3 (135.6, 6) -> (135.6, 4)
extrude "Extrude20" add sketch "Sketch20" along normal blind 25.6 from surface at 2.4 separate body makes body 40 in component "Лоток"
sketch "Sketch21" plane through (0, 0, 0) normal (0, 0, 1) x (1, 0, 0) in component "Лоток"
  line L0 (135.6, 111) -> (137.6, 111)
  line L1 (137.6, 111) -> (137.6, 113)
  line L2 (137.6, 113) -> (135.6, 113)
  line L3 (135.6, 113) -> (135.6, 111)
extrude "Extrude21" add sketch "Sketch21" along normal blind 42.6 from surface at 2.4 separate body makes body 41 in component "Лоток"
sketch "Sketch22" plane through (0, 0, 0) normal (0, 0, 1) x (1, 0, 0) in component "Лоток"
  line L0 (163.4, 4) -> (165.4, 4)
  line L1 (165.4, 4) -> (165.4, 6)
  line L2 (165.4, 6) -> (163.4, 6)
  line L3 (163.4, 6) -> (163.4, 4)
extrude "Extrude22" add sketch "Sketch22" along normal blind 25.6 from surface at 2.4 separate body makes body 42 in component "Лоток"
sketch "Sketch23" plane through (0, 0, 0) normal (0, 0, 1) x (1, 0, 0) in component "Лоток"
  line L0 (163.4, 111) -> (165.4, 111)
  line L1 (165.4, 111) -> (165.4, 113)
  line L2 (165.4, 113) -> (163.4, 113)
  line L3 (163.4, 113) -> (163.4, 111)
extrude "Extrude23" add sketch "Sketch23" along normal blind 42.6 from surface at 2.4 separate body makes body 43 in component "Лоток"
sketch "Sketch24" plane through (0, 0, 0) normal (0, 0, 1) x (1, 0, 0) in component "Лоток"
  line L0 (168.6, 4) -> (170.6, 4)
  line L1 (170.6, 4) -> (170.6, 6)
  line L2 (170.6, 6) -> (168.6, 6)
  line L3 (168.6, 6) -> (168.6, 4)
extrude "Extrude24" add sketch "Sketch24" along normal blind 25.6 from surface at 2.4 separate body makes body 44 in component "Лоток"
sketch "Sketch25" plane through (0, 0, 0) normal (0, 0, 1) x (1, 0, 0) in component "Лоток"
  line L0 (168.6, 111) -> (170.6, 111)
  line L1 (170.6, 111) -> (170.6, 113)
  line L2 (170.6, 113) -> (168.6, 113)
  line L3 (168.6, 113) -> (168.6, 111)
extrude "Extrude25" add sketch "Sketch25" along normal blind 42.6 from surface at 2.4 separate body makes body 45 in component "Лоток"
combine "Combine1''" operation add target body 21 tool bodies 22 23 24 25 26 27 28 29 30 31 32 33 34 35 36 37 38 39 40 41 42 43 44 45 in component "Лоток"
sketch "Sketch26" plane through (0, 0, 0) normal (0, 1, 0) x (1, 0, 0) in component "Лоток"
  line L0 (11.4278, -20.0215) -> (30.5722, -20.0215)
  line L1 (30.5722, -20.0215) -> (21, -36.957)
  line L2 (21, -36.957) -> (11.4278, -20.0215)
  line L3 (24.4278, -38.9785) -> (43.5722, -38.9785)
  line L4 (43.5722, -38.9785) -> (34, -22.043)
  line L5 (34, -22.043) -> (24.4278, -38.9785)
  line L6 (37.4278, -20.0215) -> (56.5722, -20.0215)
  line L7 (56.5722, -20.0215) -> (47, -36.957)
  line L8 (47, -36.957) -> (37.4278, -20.0215)
  line L9 (50.4278, -38.9785) -> (69.5722, -38.9785)
  line L10 (69.5722, -38.9785) -> (60, -22.043)
  line L11 (60, -22.043) -> (50.4278, -38.9785)
  line L12 (63.4278, -20.0215) -> (82.5722, -20.0215)
  line L13 (82.5722, -20.0215) -> (73, -36.957)
  line L14 (73, -36.957) -> (63.4278, -20.0215)
  line L15 (76.4278, -38.9785) -> (95.5722, -38.9785)
  line L16 (95.5722, -38.9785) -> (86, -22.043)
  line L17 (86, -22.043) -> (76.4278, -38.9785)
  line L18 (89.4278, -20.0215) -> (108.5722, -20.0215)
  line L19 (108.5722, -20.0215) -> (99, -36.957)
  line L20 (99, -36.957) -> (89.4278, -20.0215)
  line L21 (102.4278, -38.9785) -> (121.5722, -38.9785)
  line L22 (121.5722, -38.9785) -> (112, -22.043)
  line L23 (112, -22.043) -> (102.4278, -38.9785)
  line L24 (115.4278, -20.0215) -> (134.5722, -20.0215)
  line L25 (134.5722, -20.0215) -> (125, -36.957)
  line L26 (125, -36.957) -> (115.4278, -20.0215)
  line L27 (128.4278, -38.9785) -> (147.5722, -38.9785)
  line L28 (147.5722, -38.9785) -> (138, -22.043)
  line L29 (138, -22.043) -> (128.4278, -38.9785)
  line L30 (141.4278, -20.0215) -> (160.5722, -20.0215)
  line L31 (160.5722, -20.0215) -> (151, -36.957)
  line L32 (151, -36.957) -> (141.4278, -20.0215)
  line L33 (154.4278, -38.9785) -> (173.5722, -38.9785)
  line L34 (173.5722, -38.9785) -> (164, -22.043)
  line L35 (164, -22.043) -> (154.4278, -38.9785)
  line L36 (167.4278, -20.0215) -> (186.5722, -20.0215)
  line L37 (186.5722, -20.0215) -> (177, -36.957)
  line L38 (177, -36.957) -> (167.4278, -20.0215)
extrude "Extrude26" cut sketch "Sketch26" along normal blind 20 from surface at 108 bodies 21 in component "Лоток"
sketch "Sketch1 (4)" plane through (0, 0, 0) normal (0, 0, 1) x (1, 0, 0) in component "Планка логотипа"
  line L0 (0, 0) -> (120, 0)
  dimension "d157" = 8
  text T0 "GIVANTA MASTERS" font "Arial Black" height 8 align centre spacing 1 along the path L0 letters at x, y, angle (-0.6003, 12.3001, 0) (8.7094, 12.3001, 0) (13.0587, 12.3001, 0) (21.7626, 12.3001, 0) (30.4884, 12.3001, 0) (39.7981, 12.3001, 0) (47.869, 12.3001, 0) (56.5948, 12.3001, 0) (60.322, 12.3001, 0) (70.8704, 12.3001, 0) (79.5962, 12.3001, 0) (87.6671, 12.3001, 0) (95.7381, 12.3001, 0) (103.809, 12.3001, 0) (112.5293, 12.3001, 0)
extrude "Extrude1'''" add sketch "Sketch1 (4)" along normal blind 0.8 separate body text T0 makes body 46 at (97.377, 3.7963, 0) makes body 47 at (61.7881, 4.7003, 0) makes body 48 at (28.3147, 3.6835, 0) makes body 49 at (7.3379, 2.8704, 0) makes body 50 at (38.1974, 3.8581, 0) makes body 51 at (77.4225, 3.6835, 0) makes body 52 at (105.4879, 3.749, 0) makes body 53 at (91.2688, 4.0164, 0) makes body 54 at (54.4211, 3.6835, 0) makes body 55 at (15.5562, 3.4143, 0) makes body 56 at (10.452, 5.3333, 0) makes body 57 at (43.3997, 4.0164, 0) makes body 58 at (85.0771, 4.1947, 0) makes body 59 at (118.0102, 4.1947, 0) in component "Планка логотипа"
sketch "Sketch2 (4)" plane through (0, 0, 0) normal (0, 0, 1) x (1, 0, 0) in component "Планка логотипа"
  line L0 (-9.0873, -4.6364) -> (129.1746, -4.6364)
  line L1 (129.1746, -4.6364) -> (129.1746, 12.6364)
  line L2 (129.1746, 12.6364) -> (-9.0873, 12.6364)
  line L3 (-9.0873, 12.6364) -> (-9.0873, -4.6364)
extrude "Extrude2'''" add sketch "Sketch2 (4)" along normal blind 3 from surface at -3 separate body makes body 60 in component "Планка логотипа"
sketch "Sketch1 (5)" plane through (0, 0, 0) normal (0, 0, 1) x (1, 0, 0) in component "Перегородка"
  line L0 (0, 0) -> (2.4, 0)
  line L1 (2.4, 0) -> (2.4, 109)
  line L2 (2.4, 109) -> (0, 109)
  line L3 (0, 109) -> (0, 0)
extrude "Extrude1''''" add sketch "Sketch1 (5)" along normal blind 40 separate body makes body 61 in component "Перегородка"
sketch "Sketch1 (6)" plane through (0, 0, 0) normal (0, 0, 1) x (1, 0, 0) in component "Штанга"
  line L0 (0, 0) -> (214, 0)
  line L1 (214, 0) -> (214, 10)
  line L2 (214, 10) -> (0, 10)
  line L3 (0, 10) -> (0, 0)
extrude "Extrude1'''''" add sketch "Sketch1 (6)" along normal blind 12 separate body makes body 62 in component "Штанга"
sketch "Sketch2 (5)" plane through (0, 0, 0) normal (0, 0, 1) x (1, 0, 0) in component "Штанга"
  line L0 (-5, 2) -> (0, 2)
  line L1 (0, 2) -> (0, 8)
  line L2 (0, 8) -> (-5, 8)
  line L3 (-5, 8) -> (-5, 2)
extrude "Extrude2''''" add sketch "Sketch2 (5)" along normal blind 6 from surface at 3 separate body makes body 63 in component "Штанга"
sketch "Sketch3 (4)" plane through (0, 0, 0) normal (0, 0, 1) x (1, 0, 0) in component "Штанга"
  line L0 (214, 2) -> (219, 2)
  line L1 (219, 2) -> (219, 8)
  line L2 (219, 8) -> (214, 8)
  line L3 (214, 8) -> (214, 2)
extrude "Extrude3'''" add sketch "Sketch3 (4)" along normal blind 6 from surface at 3 separate body makes body 64 in component "Штанга"
combine "Combine1'''" operation add target body 62 tool bodies 63 64 in component "Штанга"
component "Боковина левая" placed x (1, 0, 0) y (0, 1, 0) z (0, 0, 1) at (0, 0, 0)
component "Боковина правая" placed x (1, 0, 0) y (0, 1, 0) z (0, 0, 1) at (216, 0, 0)
component "Лоток" placed x (1, 0, 0) y (0, 0.978148, 0.207912) z (0, -0.207912, 0.978148) at (14.5, 20, 15)
component "Перегородка" placed x (1, 0, 0) y (0, 0.978148, 0.207912) z (0, -0.207912, 0.978148) at (81.3, 23.4136, 18.1792)
component "Штанга" placed x (1, 0, 0) y (0, 1, 0) z (0, 0, 1) at (8, 138, 8)
component "Лоток" placed x (1, 0, 0) y (0, 0.978148, 0.207912) z (0, -0.207912, 0.978148) at (14.5, 20, 90)
component "Лоток" placed x (1, 0, 0) y (0, 0.978148, 0.207912) z (0, -0.207912, 0.978148) at (14.5, 20, 165)
component "Перегородка" placed x (1, 0, 0) y (0, 0.978148, 0.207912) z (0, -0.207912, 0.978148) at (147.3, 23.4136, 18.1792)
component "Перегородка" placed x (1, 0, 0) y (0, 0.978148, 0.207912) z (0, -0.207912, 0.978148) at (81.3, 23.4136, 93.1792)
component "Перегородка" placed x (1, 0, 0) y (0, 0.978148, 0.207912) z (0, -0.207912, 0.978148) at (147.3, 23.4136, 93.1792)
component "Перегородка" placed x (1, 0, 0) y (0, 0.978148, 0.207912) z (0, -0.207912, 0.978148) at (81.3, 23.4136, 168.1792)
component "Перегородка" placed x (1, 0, 0) y (0, 0.978148, 0.207912) z (0, -0.207912, 0.978148) at (147.3, 23.4136, 168.1792)
component "Штанга" placed x (1, 0, 0) y (0, 1, 0) z (0, 0, 1) at (8, 138, 220)
component "Планка логотипа" placed x (1, 0, 0) y (0, -0.207912, 0.978148) z (0, -0.978148, -0.207912) at (54.9563, 15.062, 173.8021)
equation "d158 = 'GIVANTA MASTERS'"
named bodies: "Тело", "Логотип (2-й цвет)", "Логотип", "Логотип (1)", "Логотип (2)", "Логотип (3)", "Логотип (4)", "Логотип (5)", "Логотип (6)", "Логотип (7)", "Логотип (8)", "Логотип (9)", "Логотип (10)", "Логотип (11)", "Логотип (12)"
